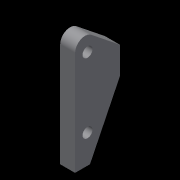
# Autodesk Inventor part: Knuckle
Saved by Autodesk Inventor 2015 (Build 190159000, 159)
## iProperties
RuleStatus: InUse
Created: 2014-10-27
Part Number: Knuckle
Material: Generic
Document SubType Name: Modeling
Designer: Inventor
Mass: 0.436768 g
Surface Area: 4.93521 cm^2
Volume: 0.436768 cm^3
Density: 1 g/cm^3
Appearance: Default
BeforeDocSave0: UpdateBoundingBox
CX: 3.00 mm
CY: 9.00 mm
CZ: 22.84 mm
Author: Inventor
Autodesk Inventor part; units mm, degrees
ref_plane "YZ Plane" through (0, 0, 0) normal (1, 0, 0) x (0, 1, 0)
ref_plane "XZ Plane" through (0, 0, 0) normal (0, 1, 0) x (-1, 0, 0)
ref_plane "XY Plane" through (0, 0, 0) normal (0, 0, 1) x (1, 0, 0)
sketch "Base" plane through (0, 0, 0) normal (1, 0, 0) x (0, 1, 0)
  line L0 (3, -25) -> (0, -25)
  line L1 (3, -25) -> (9, -12.6982)
  line L2 (9, -12.6982) -> (9, -7.1982)
  line L3 (9, -7.1982) -> (0, 0)
  line L4 (0, -25) -> (0, 0)
  dimension "d0" = 9
  dimension "d2" = 26
  dimension "d3" = 25
  dimension "d4" = 3
  dimension "d24" = 5.5
  constraints: 10 end point, 1 coincident, 1 perpendicular, 1 vertical
  measures "d0" distance between parallel lines of L2 L4
  measures "d2" angle of L1 L4
  measures "d3" distance of L0.end L3.end
  measures "d4" distance of L0.start L0.end
  measures "d24" distance of L1.end L2.end
extrude "BaseFeature" add sketch "Base" along normal blind 3
fillet "BaseFilletsFeature" radius 2 1 edges at (1.5, 0, 0)
sketch "BaseHoles" plane through (0, 0, 0) normal (-1, 0, 0) x (0, 0, 1)
  line L0 (-25, 2.5) -> (-2.2241, 2.5) construction
  line L1 (-2.5987, 3.2492) -> (-7.1982, 9) construction
  circle A0 centre (-19.2241, 2.5) radius 1.75
  circle A1 centre (-5.2241, 2.5) radius 1.75
  line L2 (-4.1606, 0) -> (-25, 0) projected
  arc A2 (-4.1606, 0) -> (-2.5987, 3.2492) centre (-4.1606, 2) ccw projected
  line L3 (-25, 0) -> (-25, 3) projected
  dimension "d9" = 3.5
  dimension "d12" = 3
  dimension "d23" = 14
  dimension "d25" = 2.5
  constraints: 3 point on line, 2 centre point, 2 end point, 1 equal radius, 1 horizontal, 1 point on circle
  measures "d9" diameter of A0
  measures "d12" distance of L0.end A1.centre
  measures "d23" distance of A0.centre A1.centre
  measures "d25" distance between parallel lines of L2 L0
hole "BaseHolesFeature" at (0, 2.5, -19.2241) at (0, 2.5, -5.2241) direction (1, 0, 0) diameter 2 end through all
body "Solid1"
